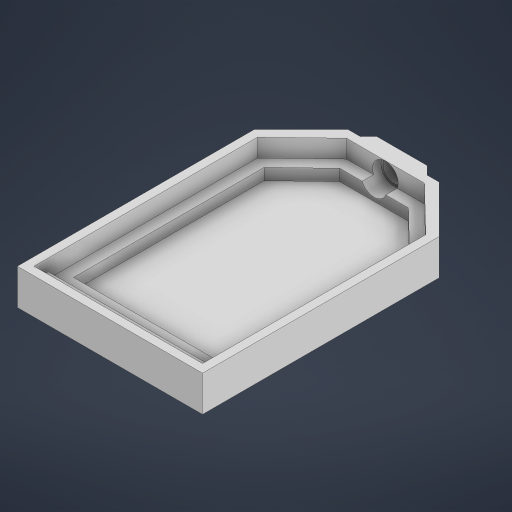
# Autodesk Inventor part: rc5_box_2
Saved by Autodesk Inventor 2024 (Build 280153000, 153)
## iProperties
Created: 2024-03-19
Part Number: rc5_box_2
Material: Všeobecné
Document SubType Name: Modeling
Designer: Simak
Density: 1 g/cm^3
Appearance: Výchozí
Author: Simak
Autodesk Inventor part; units mm, degrees
ref_plane "YZ Plane" through (0, 0, 0) normal (1, 0, 0) x (0, 1, 0)
ref_plane "XZ Plane" through (0, 0, 0) normal (0, 1, 0) x (-1, 0, 0)
ref_plane "XY Plane" through (0, 0, 0) normal (0, 0, 1) x (1, 0, 0)
sketch "Náčrt1" plane through (0, 0, 0) normal (0, 1, 0) x (-1, 0, 0)
  line L0 (20, -19.5) -> (20, 29.85) construction
  line L1 (20, 29.85) -> (-20, 29.85) construction
  line L2 (-20, 29.85) -> (-20, -19.5) construction
  line L3 (-20, -19.5) -> (-9.25, -29.85) construction
  line L4 (-9.25, -29.85) -> (9.25, -29.85) construction
  line L5 (9.25, -29.85) -> (20, -19.5) construction
  line L6 (0, 0) -> (20, 29.85) construction
  line L7 (0, 0) -> (-20, 29.85) construction
  line L8 (0, 0) -> (-20, -29.85) construction
  line L9 (-20, -29.85) -> (-9.25, -29.85) construction
  line L10 (-20, -29.85) -> (-20, -19.5)
  line L11 (17.5, -18.4366) -> (17.5, 27.35)
  line L12 (17.5, 27.35) -> (-17.5, 27.35)
  line L13 (-17.5, 27.35) -> (-17.5, -18.4366)
  line L14 (-17.5, -18.4366) -> (-8.2421, -27.35)
  line L15 (-8.2421, -27.35) -> (8.2421, -27.35)
  line L16 (8.2421, -27.35) -> (17.5, -18.4366)
  line L17 (20.25, -19.6063) -> (20.25, 30.1)
  line L18 (20.25, 30.1) -> (-20.25, 30.1)
  line L19 (-20.25, 30.1) -> (-20.25, -19.6063)
  line L20 (-20.25, -19.6063) -> (-9.3508, -30.1)
  line L21 (-9.3508, -30.1) -> (9.3508, -30.1)
  line L22 (9.3508, -30.1) -> (20.25, -19.6063)
  line L23 (22.25, -20.7863) -> (22.25, 32.1)
  line L24 (22.25, 32.1) -> (-22.25, 32.1) construction
  line L25 (-22.25, 32.1) -> (-22.25, -20.7863)
  line L26 (-22.25, -20.7863) -> (-10.9363, -32.1)
  line L27 (-10.9363, -32.1) -> (10.9363, -32.1)
  line L28 (10.9363, -32.1) -> (22.25, -20.7863)
  line L29 (20.25, 30.1) -> (20.25, 34.1)
  line L30 (20.25, 34.1) -> (-20.25, 34.1)
  line L31 (-20.25, 34.1) -> (-20.25, 30.1)
  line L32 (22.25, 32.1) -> (22.25, 36.1)
  line L33 (22.25, 36.1) -> (-22.25, 36.1)
  line L34 (-22.25, 36.1) -> (-22.25, 32.1)
  line L35 (20.25, 30.7) -> (-20.25, 30.7)
  point P0 (0, -32.1)
  dimension "d0" = 40
  dimension "d1" = 59.7
  dimension "d2" = 18.5
  dimension "d4" = 49.35
  dimension "d6" = 2.5
  dimension "d9" = 4
  dimension "d10" = 2
  dimension "d19" = 0.25
  dimension "d20" = 2
  dimension "d21" = 135
  dimension "d22" = 2
  dimension "d24" = 16
  dimension "d45" = 0.6
  constraints: 72 end point, 6 equal length, 4 horizontal, 4 perpendicular, 4 vertical, 2 point on line, 1 collinear, 1 midpoint, 1 vertical alignment, 12 other
  measures "d0" distance between parallel lines of L0 L2
  measures "d1" distance between parallel lines of L1 L4
  measures "d2" distance of L3.end L4.end
  measures "d4" distance of L1.end L2.end
  measures "d6" distance between parallel lines of L5 L16
  measures "d9" distance between parallel lines of L30 L18
  measures "d10" distance between parallel lines of L33 L30
  measures "d19" distance between parallel lines of L5 L22
  measures "d20" distance between parallel lines of L17 L23
  measures "d21" angle of L28 L23
  measures "d22" distance between parallel lines of L27 L21
  measures "d24" distance of L27.end L23.start
  measures "d45" distance between parallel lines of L18 L35
extrude "Vysunutí1" add sketch "Náčrt1" along normal blind 1.5 contours L16 L15 L14 L13 L12 L11 | L22 L21 L20 L19 L18 L17 | L18 L31 L35 L29 | L35 L31 L30 L29 | L28 L27 L26 L25 L34 L33 L32 L23
extrude "Vysunutí2" add sketch "Náčrt1" along normal blind 4.25 contours L22 L21 L20 L19 L18 L17 | L18 L31 L35 L29
extrude "Vysunutí3" add sketch "Náčrt1" along normal blind 5.75 contours L35 L31 L30 L29
extrude "Vysunutí4" add sketch "Náčrt1" along normal blind 8.58 contours L28 L27 L26 L25 L34 L33 L32 L23
sketch "Náčrt2" plane through (0, 0, 0) normal (0, -1, 0) x (1, 0, 0)
  line L0 (10.9363, -32.1) -> (-10.9363, -32.1) projected
  line L1 (22.25, -20.7863) -> (10.9363, -32.1) projected
  line L2 (22.25, 36.1) -> (22.25, -20.7863) projected
  line L3 (-22.25, 36.1) -> (22.25, 36.1) projected
  line L4 (-22.25, -20.7863) -> (-22.25, 36.1) projected
  line L5 (-10.9363, -32.1) -> (-22.25, -20.7863) projected
  line L6 (8, -32.1) -> (6, -34.1)
  line L7 (6, -34.1) -> (-6, -34.1)
  line L8 (-6, -34.1) -> (-8, -32.1)
  line L9 (10.9363, -32.1) -> (-10.9363, -32.1) projected
  line L10 (10.9363, -32.1) -> (6, -34.1) construction
  line L11 (-6, -34.1) -> (-10.9363, -32.1) construction
  point P0 (0, 0)
  dimension "d25" = 45
  dimension "d26" = 2
  dimension "d27" = 12
  constraints: 10 end point, 2 point on line, 1 equal length, 1 horizontal, 1 perpendicular
  measures "d25" angle of L0 L6
  measures "d26" distance between parallel lines of L0 L7
  measures "d27" distance of L6.end L7.end
extrude "Vysunutí5" add sketch "Náčrt2" against normal up to surface (8.58 mm away) contours L6 L7 L8 L0
sketch "Náčrt3" plane through (-9.3508, 4.25, -30.1) normal (0, 0, 1) x (1, 0, 0)
  line L0 (18.7016, 0) -> (0, 0) projected
  line L1 (18.7016, 0) -> (18.7016, 4.33) projected
  line L2 (0, 4.33) -> (18.7016, 4.33) projected
  line L3 (0, 0) -> (0, 4.33) projected
  line L4 (17.5929, -2.75) -> (1.1087, -2.75) projected
  line L5 (17.5929, -2.75) -> (17.5929, 0) projected
  line L6 (1.1087, 0) -> (17.5929, 0) projected
  line L7 (1.1087, -2.75) -> (1.1087, 0) projected
  circle A0 centre (9.3508, 1.175) radius 3.075
  line L8 (3.3508, 4.33) -> (15.3508, 4.33) projected
  line L9 (15.3508, -4.25) -> (15.3508, 4.33) projected
  line L10 (3.3508, -4.25) -> (15.3508, -4.25) projected
  line L11 (3.3508, -4.25) -> (3.3508, 4.33) projected
  line L12 (29.6008, 1.5) -> (-10.8992, 1.5) projected
  point P0 (9.3508, -4.25)
  point P1 (29.6008, 0.83)
  point P2 (-10.8992, 0.83)
  point P3 (9.3508, 4.33)
  point P4 (9.3508, 1.5)
  point P5 (9.3508, 4.33)
  point P6 (9.3508, 0)
  point P7 (9.3508, -2.75)
  point P8 (-10.8992, 1.5)
  dimension "d31" = 6.15
  dimension "d46" = 2.75
  constraints: 4 midpoint, 4 vertical alignment, 1 centre point, 2 other
  measures "d31" diameter of A0
extrude "Vysunutí6" cut sketch "Náčrt3" along normal blind 7 and the other way blind 2 contours A0 L0 | L0 A0 L12 | L12 A0
sketch "Náčrt4" plane through (0, 5.425, -32.1) normal (0, 0, 1) x (1, 0, 0)
  circle A0 centre (0, 0) radius 3.075 projected
  point P0 (0, -5.425)
  point P1 (-1.4433, 2.63)
  point P2 (1.4433, 2.63)
  point P3 (-1.199, 2.75)
  point P4 (1.199, 2.75)
  constraints: 1 coincident, 1 other
hole "Díra1" at (0, 5.425, -32.1) direction (0, 0, -1) diameter 5.15 end through all
equation "\"d10\" = d8"
equation "\"d8\" = 2"
